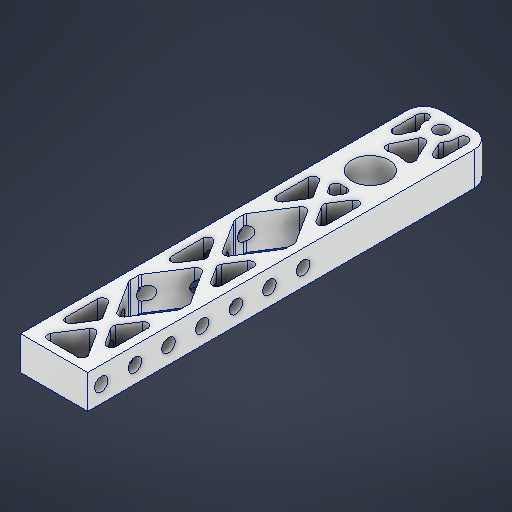
# Autodesk Inventor part: climber-arm-middle-bar
Saved by Autodesk Inventor 2025.1 (Build 291241020, 241B)
## iProperties
Created: 2025-03-18
Part Number: climber-arm-middle-bar
Material: Aluminum 6061
Document SubType Name: Modeling
Designer: mathe
Density: 2.7 g/cm^3
Appearance: Aluminum - Flat
Author: mathe
Autodesk Inventor part; units mm, degrees
ref_plane "YZ Plane" through (0, 0, 0) normal (1, 0, 0) x (0, 1, 0)
ref_plane "XZ Plane" through (0, 0, 0) normal (0, 1, 0) x (-1, 0, 0)
ref_plane "XY Plane" through (0, 0, 0) normal (0, 0, 1) x (1, 0, 0)
sketch "Sketch1" plane through (0, 0, 0) normal (0, 1, 0) x (-1, 0, 0)
  line L0 (6.35, -152.4) -> (19.05, -152.4)
  arc A0 (19.05, -152.4) -> (25.4, -146.05) centre (19.05, -146.05) ccw
  line L1 (25.4, -146.05) -> (25.4, 0)
  line L2 (25.4, 0) -> (0, 0)
  line L3 (0, 0) -> (0, -146.05)
  arc A1 (0, -146.05) -> (6.35, -152.4) centre (6.35, -146.05) ccw
  arc A2 (9.5889, -129.0519) -> (15.8111, -129.0519) centre (12.7, -119.38) ccw
  arc A3 (17.8994, -131.4388) -> (15.8111, -129.0519) centre (16.34, -130.6962) ccw
  line L4 (17.8994, -131.4388) -> (14.2594, -139.0828)
  arc A4 (11.1406, -139.0828) -> (14.2594, -139.0828) centre (12.7, -138.3402) ccw
  line L5 (11.1406, -139.0828) -> (7.5006, -131.4388)
  arc A5 (9.5889, -129.0519) -> (7.5006, -131.4388) centre (9.06, -130.6962) ccw
  line L6 (10.2235, -60.6193) -> (6.3581, -66.6751)
  arc A6 (3.175, -65.7458) -> (6.3581, -66.6751) centre (4.9022, -65.7458) ccw
  line L7 (3.175, -65.7458) -> (3.175, -53.6342)
  arc A7 (6.3581, -52.7049) -> (3.175, -53.6342) centre (4.9022, -53.6342) ccw
  line L8 (6.3581, -52.7049) -> (10.2235, -58.7607)
  arc A8 (10.2235, -60.6193) -> (10.2235, -58.7607) centre (8.7676, -59.69) ccw
  line L9 (22.225, -38.274) -> (22.225, -41.3127)
  arc A9 (21.9537, -42.242) -> (22.225, -41.3127) centre (20.4978, -41.3127) ccw
  line L10 (21.9537, -42.242) -> (14.1559, -54.4585)
  arc A10 (11.2441, -54.4585) -> (14.1559, -54.4585) centre (12.7, -53.5293) ccw
  line L11 (11.2441, -54.4585) -> (3.4463, -42.242)
  arc A11 (3.175, -41.3127) -> (3.4463, -42.242) centre (4.9022, -41.3127) ccw
  line L12 (3.175, -41.3127) -> (3.175, -38.274)
  arc A12 (3.4463, -37.3447) -> (3.175, -38.274) centre (4.9022, -38.274) ccw
  line L13 (3.4463, -37.3447) -> (11.2441, -25.1281)
  arc A13 (14.1559, -25.1281) -> (11.2441, -25.1281) centre (12.7, -26.0574) ccw
  line L14 (14.1559, -25.1281) -> (21.9537, -37.3447)
  arc A14 (22.225, -38.274) -> (21.9537, -37.3447) centre (20.4978, -38.274) ccw
  line L15 (22.225, -53.6342) -> (22.225, -65.7458)
  arc A15 (19.0419, -66.6751) -> (22.225, -65.7458) centre (20.4978, -65.7458) ccw
  line L16 (19.0419, -66.6751) -> (15.1765, -60.6193)
  arc A16 (15.1765, -58.7607) -> (15.1765, -60.6193) centre (16.6324, -59.69) ccw
  line L17 (15.1765, -58.7607) -> (19.0419, -52.7049)
  arc A17 (22.225, -53.6342) -> (19.0419, -52.7049) centre (20.4978, -53.6342) ccw
  line L18 (15.1765, -18.9674) -> (19.0419, -12.9116)
  arc A18 (22.225, -13.8409) -> (19.0419, -12.9116) centre (20.4978, -13.8409) ccw
  line L19 (22.225, -13.8409) -> (22.225, -25.9525)
  arc A19 (19.0419, -26.8818) -> (22.225, -25.9525) centre (20.4978, -25.9525) ccw
  line L20 (19.0419, -26.8818) -> (15.1765, -20.826)
  arc A20 (15.1765, -18.9674) -> (15.1765, -20.826) centre (16.6324, -19.8967) ccw
  line L21 (14.1559, -104.7148) -> (15.376, -106.6263)
  arc A21 (13.7428, -109.2737) -> (15.376, -106.6263) centre (13.9201, -107.5556) ccw
  arc A22 (13.7428, -109.2737) -> (11.6572, -109.2737) centre (12.7, -119.38) ccw
  arc A23 (10.024, -106.6263) -> (11.6572, -109.2737) centre (11.4799, -107.5556) ccw
  line L22 (10.024, -106.6263) -> (11.2441, -104.7148)
  arc A24 (14.1559, -104.7148) -> (11.2441, -104.7148) centre (12.7, -105.6441) ccw
  line L23 (22.225, -78.0673) -> (22.225, -81.106)
  arc A25 (21.9537, -82.0353) -> (22.225, -81.106) centre (20.4978, -81.106) ccw
  line L24 (21.9537, -82.0353) -> (14.1559, -94.2519)
  arc A26 (11.2441, -94.2519) -> (14.1559, -94.2519) centre (12.7, -93.3226) ccw
  line L25 (11.2441, -94.2519) -> (3.4463, -82.0353)
  arc A27 (3.175, -81.106) -> (3.4463, -82.0353) centre (4.9022, -81.106) ccw
  line L26 (3.175, -81.106) -> (3.175, -78.0673)
  arc A28 (3.4463, -77.138) -> (3.175, -78.0673) centre (4.9022, -78.0673) ccw
  line L27 (3.4463, -77.138) -> (11.2441, -64.9215)
  arc A29 (14.1559, -64.9215) -> (11.2441, -64.9215) centre (12.7, -65.8507) ccw
  line L28 (14.1559, -64.9215) -> (21.9537, -77.138)
  arc A30 (22.225, -78.0673) -> (21.9537, -77.138) centre (20.4978, -78.0673) ccw
  line L29 (15.1765, -98.554) -> (19.0419, -92.4982)
  arc A31 (22.225, -93.4275) -> (19.0419, -92.4982) centre (20.4978, -93.4275) ccw
  line L30 (22.225, -93.4275) -> (22.225, -105.5391)
  arc A32 (19.0419, -106.4684) -> (22.225, -105.5391) centre (20.4978, -105.5391) ccw
  line L31 (19.0419, -106.4684) -> (15.1765, -100.4126)
  arc A33 (15.1765, -98.554) -> (15.1765, -100.4126) centre (16.6324, -99.4833) ccw
  line L32 (10.2235, -20.826) -> (6.3581, -26.8818)
  arc A34 (3.175, -25.9525) -> (6.3581, -26.8818) centre (4.9022, -25.9525) ccw
  line L33 (3.175, -25.9525) -> (3.175, -13.8409)
  arc A35 (6.3581, -12.9116) -> (3.175, -13.8409) centre (4.9022, -13.8409) ccw
  line L34 (6.3581, -12.9116) -> (10.2235, -18.9674)
  arc A36 (10.2235, -20.826) -> (10.2235, -18.9674) centre (8.7676, -19.8967) ccw
  arc A37 (7.0615, -3.175) -> (5.6056, -5.8315) centre (7.0615, -4.9022) ccw
  line L35 (7.0615, -3.175) -> (18.3385, -3.175)
  arc A38 (19.7944, -5.8315) -> (18.3385, -3.175) centre (18.3385, -4.9022) ccw
  line L36 (19.7944, -5.8315) -> (14.1559, -14.6652)
  arc A39 (11.2441, -14.6652) -> (14.1559, -14.6652) centre (12.7, -13.7359) ccw
  line L37 (11.2441, -14.6652) -> (5.6056, -5.8315)
  arc A40 (17.0041, -140.7037) -> (17.2051, -142.5129) centre (18.5636, -141.4463) ccw
  line L38 (17.0041, -140.7037) -> (18.9384, -136.6418)
  arc A41 (22.225, -137.3844) -> (18.9384, -136.6418) centre (20.4978, -137.3844) ccw
  line L39 (22.225, -137.3844) -> (22.225, -146.05)
  arc A42 (21.3219, -148.2679) -> (22.225, -146.05) centre (19.05, -146.05) ccw
  arc A43 (18.3747, -146.8271) -> (21.3219, -148.2679) centre (20.086, -147.0614) ccw
  arc A44 (18.3747, -146.8271) -> (17.2051, -142.5129) centre (12.7, -146.05) ccw
  line L40 (3.175, -146.05) -> (3.175, -137.3844)
  arc A45 (6.4616, -136.6418) -> (3.175, -137.3844) centre (4.9022, -137.3844) ccw
  line L41 (6.4616, -136.6418) -> (8.3959, -140.7037)
  arc A46 (8.1949, -142.5129) -> (8.3959, -140.7037) centre (6.8364, -141.4463) ccw
  arc A47 (8.1949, -142.5129) -> (7.0253, -146.8271) centre (12.7, -146.05) ccw
  arc A48 (4.0781, -148.2679) -> (7.0253, -146.8271) centre (5.314, -147.0614) ccw
  arc A49 (3.175, -146.05) -> (4.0781, -148.2679) centre (6.35, -146.05) ccw
  line L42 (10.2235, -100.4126) -> (6.3581, -106.4684)
  arc A50 (3.175, -105.5391) -> (6.3581, -106.4684) centre (4.9022, -105.5391) ccw
  line L43 (3.175, -105.5391) -> (3.175, -93.4275)
  arc A51 (6.3581, -92.4982) -> (3.175, -93.4275) centre (4.9022, -93.4275) ccw
  line L44 (6.3581, -92.4982) -> (10.2235, -98.554)
  arc A52 (10.2235, -100.4126) -> (10.2235, -98.554) centre (8.7676, -99.4833) ccw
  circle A53 centre (12.7, -119.38) radius 6.985
  circle A54 centre (12.7, -146.05) radius 2.5527
  point P0 (25.4, -146.05)
  point P1 (6.3581, -92.4982)
  point P2 (8.1949, -142.5129)
  point P3 (7.0253, -146.8271)
  point P4 (21.3219, -148.2679)
  point P5 (18.3747, -146.8271)
  point P6 (17.2051, -142.5129)
  point P7 (17.0041, -140.7037)
  point P8 (6.3581, -12.9116)
  point P9 (22.225, -93.4275)
  point P10 (21.9537, -82.0353)
  point P11 (11.2441, -94.2519)
  point P12 (3.4463, -82.0353)
  point P13 (3.175, -81.106)
  point P14 (3.4463, -77.138)
  point P15 (10.024, -106.6263)
  point P16 (13.7428, -109.2737)
  point P17 (15.1765, -58.7607)
  point P18 (11.2441, -54.4585)
  point P19 (3.175, -41.3127)
  point P20 (3.4463, -37.3447)
  point P21 (17.8994, -131.4388)
  constraints: 106 point on circle, 90 end point, 55 centre point
extrude "Extrusion1" add sketch "Sketch1" along normal blind 12.7
sketch "Sketch2" plane through (-25.4, 0, -146.05) normal (-1, 0, 0) x (0, 0, 1)
  line L0 (146.05, 0) -> (146.05, 12.7) projected
  line L1 (146.05, 6.35) -> (140.97, 6.35)
  point P0 (128.27, 6.35)
  point P1 (115.57, 6.35)
  point P2 (102.87, 6.35)
  point P3 (90.17, 6.35)
  point P4 (77.47, 6.35)
  point P5 (64.77, 6.35)
  dimension "d2" = 5.08
  dimension "d5" = 12.7
  constraints: 2 end point, 2 horizontal, 1 coincident, 1 midpoint, 6 other
  measures "d2" distance of L1.start L1.end
  measures "d5" distance of point (140.97, 6.35) point (128.27, 6.35)
hole "Hole1" at (-25.4, 6.35, -5.08) at (-25.4, 6.35, -17.78) at (-25.4, 6.35, -30.48) at (-25.4, 6.35, -43.18) at (-25.4, 6.35, -55.88) at (-25.4, 6.35, -68.58) at (-25.4, 6.35, -81.28) direction (1, 0, 0) diameter 5.1054 end through all
body "Solid1"
